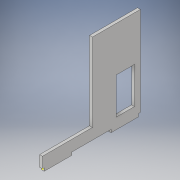
# Autodesk Inventor part: rib
Saved by Autodesk Inventor 2019 (Build 230136000, 136)
## iProperties
Created: 2018-09-07
Part Number: rib
Material: Generic
Document SubType Name: Modeling
Designer: mspet
Density: 1 g/cm^3
Appearance: Default
Author: mspet
Autodesk Inventor part; units mm, degrees
ref_plane "YZ Plane" through (0, 0, 0) normal (1, 0, 0) x (0, 1, 0)
ref_plane "XZ Plane" through (0, 0, 0) normal (0, 1, 0) x (-1, 0, 0)
ref_plane "XY Plane" through (0, 0, 0) normal (0, 0, 1) x (1, 0, 0)
sketch "Sketch1" plane through (0, 0, 0) normal (1, 0, 0) x (0, 1, 0)
  line L0 (0, 0) -> (98.425, 0)
  line L1 (98.425, 0) -> (98.425, -107.95)
  line L2 (98.425, -107.95) -> (0, -107.95)
  line L3 (0, -107.95) -> (0, 0)
  line L4 (0, -1.905) -> (-3.175, -1.905)
  line L5 (-3.175, -1.905) -> (-3.175, -32.385)
  line L6 (-3.175, -32.385) -> (0, -32.385)
  line L7 (0, -32.385) -> (0, -1.905)
  line L8 (0, -75.565) -> (-3.175, -75.565)
  line L9 (-3.175, -75.565) -> (-3.175, -106.045)
  line L10 (-3.175, -106.045) -> (0, -106.045)
  line L11 (0, -106.045) -> (0, -75.565)
  dimension "d0" = 107.95
  dimension "d1" = 3.175
  dimension "d2" = 3.175
  dimension "d3" = 30.48
  dimension "d4" = 30.48
  dimension "d5" = 1.905
  dimension "d6" = 1.905
  dimension "d7" = 98.425
  constraints: 24 end point, 6 parallel, 3 horizontal, 3 perpendicular, 2 point on line
  measures "d0" distance of L2.end L0.start
  measures "d1" distance of L5.end L6.end
  measures "d2" distance of L9.end L10.end
  measures "d3" distance of L8.end L9.end
  measures "d4" distance of L4.end L5.end
  measures "d5" distance between parallel lines of L0 L4
  measures "d6" distance between parallel lines of L2 L10
  measures "d7" distance of L1.end L2.end
extrude "Extrusion1" add sketch "Sketch1" along normal blind 3.175
sketch "Sketch2" plane through (3.175, 0, 0) normal (1, 0, 0) x (0, 0, -1)
  line L0 (101.6, 49.149) -> (81.28, 49.149)
  line L1 (81.28, 49.149) -> (81.28, 8.89)
  line L2 (81.28, 8.89) -> (101.6, 8.89)
  line L3 (101.6, 8.89) -> (101.6, 49.149)
  line L4 (32.385, 0) -> (75.565, 0) projected
  line L5 (0, 98.425) -> (0, 0) projected
  line L6 (107.95, 0) -> (107.95, 98.425) projected
  dimension "d10" = 40.259
  dimension "d11" = 20.32
  dimension "d12" = 8.89
  dimension "d14" = 6.35
  constraints: 8 end point, 2 parallel, 1 horizontal, 1 perpendicular
  measures "d10" distance of L2.end L0.start
  measures "d11" distance of L1.end L2.end
  measures "d12" distance between parallel lines of L4 L2
  measures "d14" distance between parallel lines of L6 L3
extrude "Extrusion2" cut sketch "Sketch2" against normal blind 3.175
sketch "Sketch3" plane through (3.175, 0, 0) normal (1, 0, 0) x (0, 0, -1)
  point P0 (0, 0)
sketch "Sketch4" plane through (3.175, 0, 0) normal (1, 0, 0) x (0, 0, -1)
  line L0 (-26.3959, 105.0556) -> (55.1146, 105.0556)
  line L1 (55.1146, 105.0556) -> (55.1146, 12.1421)
  line L2 (55.1146, 12.1421) -> (-26.3959, 12.1421)
  line L3 (-26.3959, 12.1421) -> (-26.3959, 105.0556)
  point P0 (0, 0)
  constraints: 8 end point, 2 parallel, 1 horizontal, 1 perpendicular
extrude "Extrusion3" cut sketch "Sketch4" against normal blind 3.175
body "Solid1"
